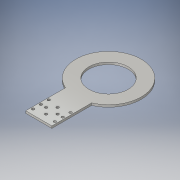
# Autodesk Inventor part: goniometer_stage_top_v1
Saved by Autodesk Inventor 2016 (Build 200138000, 138)
## iProperties
Created: 2017-01-09
Part Number: goniometer_stage_top_v1
Material: Stainless Steel AISI 304
Document SubType Name: Modeling
Designer: stephenholtz
Density: 8 g/cm^3
Appearance: Chrome - Satin
Author: stephenholtz
Autodesk Inventor part; units mm, degrees
ref_plane "YZ Plane" through (0, 0, 0) normal (1, 0, 0) x (0, 1, 0)
ref_plane "XZ Plane" through (0, 0, 0) normal (0, 1, 0) x (-1, 0, 0)
ref_plane "XY Plane" through (0, 0, 0) normal (0, 0, 1) x (1, 0, 0)
sketch "Sketch1" plane through (0, 0, 0) normal (0, 0, 1) x (1, 0, 0)
  line L0 (19.05, -19.05) -> (-19.05, -19.05)
  line L1 (-19.05, -19.05) -> (-19.05, 19.05)
  line L2 (-19.05, 19.05) -> (19.05, 19.05)
  line L3 (19.05, 19.05) -> (19.05, -19.05)
  line L4 (19.05, -19.05) -> (-19.05, 19.05) construction
  line L5 (-19.05, -19.05) -> (19.05, 19.05) construction
  line L6 (-19.05, 19.05) -> (19.05, 19.05)
  line L7 (19.05, 19.05) -> (19.05, 44.45)
  line L8 (19.05, 44.45) -> (-19.05, 44.45)
  line L9 (-19.05, 44.45) -> (-19.05, 19.05)
  line L10 (0, 19.05) -> (0, 82.55)
  circle A0 centre (0, 82.55) radius 47.625
  circle A1 centre (0, 82.55) radius 28.575
  point P0 (0, 0)
  dimension "d0" = 38.1
  dimension "d1" = 38.1
  dimension "d2" = 25.4
  dimension "d3" = 63.5
  dimension "d4" = 95.25
  dimension "d5" = 57.15
  constraints: 22 end point, 4 parallel, 3 midpoint, 2 centre point, 2 coincident, 2 horizontal, 2 perpendicular, 1 vertical
  measures "d0" distance of L1.end L2.end
  measures "d1" distance of L0.end L1.end
  measures "d2" distance of L2.end L7.end
  measures "d3" distance of L10.start L10.end
  measures "d4" diameter of A0
  measures "d5" diameter of A1
extrude "Extrusion1" add sketch "Sketch1" along normal blind 3.175
sketch "Sketch2" plane through (0, 0, 3.175) normal (0, 0, 1) x (1, 0, 0)
  circle A0 centre (0, 82.55) radius 28.575 construction
  arc A1 (19.05, 38.901) -> (-19.05, 38.901) centre (0, 82.55) ccw construction
  line L0 (-19.05, 38.901) -> (-19.05, -19.05) construction
  line L1 (-19.05, -19.05) -> (19.05, -19.05) construction
  line L2 (19.05, -19.05) -> (19.05, 38.901) construction
  line L3 (-19.05, -19.05) -> (19.05, -19.05) construction
  line L4 (19.05, -19.05) -> (19.05, 19.05) construction
  line L5 (19.05, 19.05) -> (-19.05, 19.05) construction
  line L6 (-19.05, 19.05) -> (-19.05, -19.05) construction
  line L7 (15.875, -11.43) -> (-15.875, -11.43) construction
  line L8 (-15.875, -11.43) -> (-15.875, 11.43) construction
  line L9 (-15.875, 11.43) -> (15.875, 11.43) construction
  line L10 (15.875, 11.43) -> (15.875, -11.43) construction
  line L11 (15.875, -11.43) -> (-15.875, 11.43) construction
  line L12 (-15.875, -11.43) -> (15.875, 11.43) construction
  line L13 (11.43, -15.875) -> (-11.43, -15.875) construction
  line L14 (-11.43, -15.875) -> (-11.43, 15.875) construction
  line L15 (-11.43, 15.875) -> (11.43, 15.875) construction
  line L16 (11.43, 15.875) -> (11.43, -15.875) construction
  line L17 (11.43, -15.875) -> (-11.43, 15.875) construction
  line L18 (-11.43, -15.875) -> (11.43, 15.875) construction
  line L19 (0, -8.4414) -> (8.4414, 0) construction
  line L20 (8.4414, 0) -> (0, 8.4414) construction
  line L21 (0, 8.4414) -> (-8.4414, 0) construction
  line L22 (-8.4414, 0) -> (0, -8.4414) construction
  line L23 (-5.969, -5.969) -> (5.969, 5.969) construction
  line L24 (5.969, -5.969) -> (-5.969, 5.969) construction
  line L25 (-8.4414, -8.4414) -> (8.4414, -8.4414) construction
  line L26 (8.4414, -8.4414) -> (8.4414, 8.4414) construction
  line L27 (8.4414, 8.4414) -> (-8.4414, 8.4414) construction
  line L28 (-8.4414, 8.4414) -> (-8.4414, -8.4414) construction
  line L29 (-8.4414, -8.4414) -> (8.4414, 8.4414) construction
  line L30 (8.4414, -8.4414) -> (-8.4414, 8.4414) construction
  point P0 (0, 0)
  point P1 (0, 8.4414)
  point P2 (8.4414, 0)
  point P3 (-15.875, 0)
  point P4 (15.875, 0)
  dimension "d8" = 38.1
  dimension "d9" = 38.1
  dimension "d10" = 31.75
  dimension "d11" = 22.86
  dimension "d12" = 22.86
  dimension "d13" = 31.75
  dimension "d14" = 11.938
  dimension "d15" = 11.938
  dimension "d16" = 16.8829
  dimension "d17" = 16.8829
  dimension "d18" = 4.445
  dimension "d19" = 7.4336
  dimension "d20" = 5.969
  dimension "d21" = 5.969
  dimension "d22" = 4.445
  dimension "d23" = 7.4336
  dimension "d24" = 9.906
  dimension "d25" = 9.906
  dimension "d26" = 21.844
  dimension "d27" = 21.844
  dimension "d28" = 3.175
  dimension "d29" = 27.4914
  constraints: 56 end point, 12 parallel, 8 coincident, 5 perpendicular, 4 horizontal, 4 midpoint, 3 point on line
  measures "d8" distance of L5.end L4.end
  measures "d9" distance of L4.end L3.end
  measures "d10" distance of L8.end L10.start
  measures "d11" distance of L8.start L8.end
  measures "d12" distance of L15.start L15.end
  measures "d13" distance of L13.end L15.start
  measures "d14" distance of L22.start L21.start
  measures "d15" distance of L21.start L20.start
  measures "d16" distance between parallel lines of L25 L27
  measures "d17" distance between parallel lines of L28 L26
  measures "d18" distance between parallel lines of L10 L16
  measures "d19" distance between parallel lines of L10 L26
  measures "d20" distance between parallel lines of L24 L20
  measures "d21" distance between parallel lines of L23 L19
  measures "d22" distance between parallel lines of L9 L15
  measures "d23" distance between parallel lines of L15 L27
  measures "d24" distance from line of L23.end L10
  measures "d25" distance from line of L24.start L10
  measures "d26" distance from line of L24.end L10
  measures "d27" distance from line of L23.start L10
  measures "d28" distance between parallel lines of L2 L10
  measures "d29" distance between parallel lines of L1 L27
hole "Hole1" at (-15.875, 11.43, 3.175) at (-15.875, 0, 3.175) at (-15.875, -11.43, 3.175) at (15.875, -11.43, 3.175) at (15.875, 0, 3.175) at (15.875, 11.43, 3.175) at (0, 8.4414, 3.175) at (0, -8.4414, 3.175) at (8.4414, 0, 3.175) at (-8.4414, 0, 3.175) direction (0, 0, -1) diameter 3.7973 end through all
body "Solid1"
